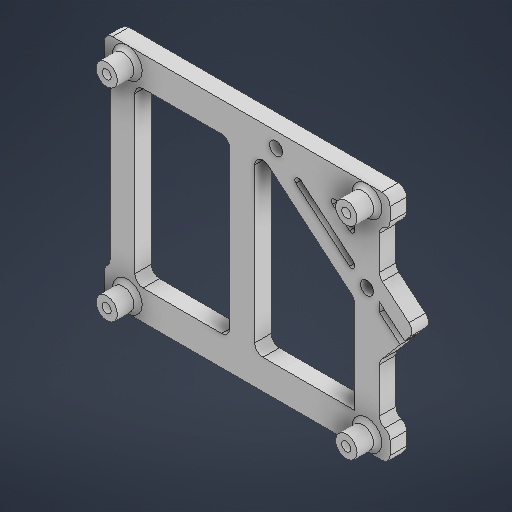
# Autodesk Inventor part: rpi-mount
Saved by Autodesk Inventor 2025 (Build 290162000, 162)
## iProperties
Created: 2024-09-27
Part Number: rpi-mount
Material: Generic
Document SubType Name: Modeling
Designer: Windows 7 was better
Density: 1 g/cm^3
Appearance: Default
Author: Windows 7 was better
Autodesk Inventor part; units mm, degrees
ref_plane "YZ Plane" through (0, 0, 0) normal (1, 0, 0) x (0, 1, 0)
ref_plane "XZ Plane" through (0, 0, 0) normal (0, 1, 0) x (-1, 0, 0)
ref_plane "XY Plane" through (0, 0, 0) normal (0, 0, 1) x (1, 0, 0)
sketch "Sketch1" plane through (0, 0, 0) normal (0, 0, 1) x (1, 0, 0)
  line L0 (0, 0) -> (0, 1.8) construction
  line L1 (-9.2123, 0.9) -> (-9.2123, 25.4) construction
  line L2 (-9.2123, 25.4) -> (-9.2123, -23.6) construction
  line L3 (-9.2123, -23.6) -> (48.7877, -23.6) construction
  line L4 (-9.2123, 25.4) -> (48.7877, 25.4) construction
  circle A0 centre (48.7877, 25.4) radius 1.1
  circle A1 centre (-9.2123, 25.4) radius 1.1
  circle A2 centre (-9.2123, -23.6) radius 1.1
  circle A3 centre (48.7877, -23.6) radius 1.1
  line L5 (-14.8123, -20) -> (54.3877, -20)
  line L6 (54.3877, -20) -> (54.3877, -27.2)
  line L7 (54.3877, -27.2) -> (-14.8123, -27.2)
  line L8 (-14.8123, -27.2) -> (-14.8123, -20)
  line L9 (-14.8123, -20) -> (54.3877, -27.2) construction
  line L10 (54.3877, -20) -> (-14.8123, -27.2) construction
  line L11 (-14.8123, 29) -> (54.3877, 29)
  line L12 (54.3877, 29) -> (54.3877, 21.8)
  line L13 (54.3877, 21.8) -> (-14.8123, 21.8)
  line L14 (-14.8123, 21.8) -> (-14.8123, 29)
  line L15 (-14.8123, 29) -> (54.3877, 21.8) construction
  line L16 (54.3877, 29) -> (-14.8123, 21.8) construction
  line L17 (21.5942, 21.8) -> (15.5942, 21.8)
  line L18 (15.5942, 21.8) -> (15.5942, -20)
  line L19 (15.5942, -20) -> (21.5942, -20)
  line L20 (21.5942, -20) -> (21.5942, 21.8)
  line L21 (-13.4058, 21.8) -> (-7.4058, 21.8)
  line L22 (-7.4058, 21.8) -> (-7.4058, -20)
  line L23 (-7.4058, -20) -> (-13.4058, -20)
  line L24 (-13.4058, -20) -> (-13.4058, 21.8)
  line L25 (19.7877, 25.4) -> (19.7877, 0) construction
  line L26 (48.7877, 25.4) -> (48.7877, -23.6) construction
  line L27 (51.7877, 25.4) -> (51.7877, -23.6)
  line L28 (51.7877, -23.6) -> (45.7877, -23.6)
  line L29 (45.7877, -23.6) -> (45.7877, 25.4)
  line L30 (45.7877, 25.4) -> (51.7877, 25.4)
  line L31 (51.7877, 25.4) -> (45.7877, -23.6) construction
  line L32 (51.7877, -23.6) -> (45.7877, 25.4) construction
  line L33 (54.2512, -3.7837) -> (27.4397, 18.7139)
  line L34 (27.4397, 18.7139) -> (30.0108, 21.7781)
  line L35 (30.0108, 21.7781) -> (56.8224, -0.7195)
  line L36 (56.8224, -0.7195) -> (54.2512, -3.7837)
  line L37 (54.2512, -3.7837) -> (89.2512, -3.7837) construction
  line L38 (30.0108, 21.7781) -> (31.1036, 23.0804) construction
  line L39 (31.1036, 23.0804) -> (57.9151, 0.5828)
  line L40 (57.9151, 0.5828) -> (60.4863, 3.647)
  line L41 (60.4863, 3.647) -> (33.6747, 26.1445)
  line L42 (33.6747, 26.1445) -> (31.1036, 23.0804)
  line L43 (54.2512, -3.7837) -> (45.7877, 3.3181)
  line L44 (47.4017, 0) -> (57.4017, 0) construction
  line L45 (56.8224, -0.7195) -> (57.9151, 0.5828) construction
  line L46 (27.4397, 18.7139) -> (23.7618, 21.8)
  line L47 (54.2512, -3.7837) -> (51.7877, -6.7196)
  line L48 (30.0108, 21.7781) -> (29.9847, 21.8)
  circle A4 centre (48.7877, 7.132) radius 1.6
  circle A5 centre (26.7826, 25.4) radius 1.6
  point P0 (19.7877, -23.6)
  point P1 (15.5942, 21.8)
  point P2 (-13.4058, -20)
  point P3 (21.5942, -20)
  point P4 (48.7877, 0.9)
  point P5 (45.7877, 21.8)
  point P6 (45.7877, -20)
  point P7 (51.7877, -20)
  point P8 (51.7877, 21.8)
  point P9 (45.7877, 15.9806)
  point P10 (38.8523, 21.8)
  point P11 (32.6294, 21.8)
  point P12 (45.7877, 10.7589)
  point P13 (45.7877, 8.5397)
  point P14 (21.5942, 20.2921)
  point P15 (21.5942, 15.0705)
  point P16 (51.7877, 3.5051)
  point P17 (51.7877, -1.7165)
  point P18 (47.6877, -23.6)
  point P19 (49.8877, -23.6)
  point P20 (51.7877, -1.7165)
  point P21 (51.7877, 5.7243)
  point P22 (51.7877, 10.946)
  point P23 (49.8877, 25.4)
  point P24 (47.6877, 25.4)
  dimension "d7" = 24.5
  dimension "d8" = 49
  dimension "d9" = 58
  dimension "d10" = 58
  dimension "d11" = 2.2
  dimension "d12" = 2.2
  dimension "d13" = 2.2
  dimension "d14" = 2.2
  dimension "d15" = 69.2
  dimension "d16" = 7.2
  dimension "d17" = 69.2
  dimension "d18" = 7.2
  dimension "d19" = 6
  dimension "d20" = 6
  dimension "d36" = 6
  dimension "d37" = 35
  dimension "d38" = 140
  dimension "d39" = 4
  dimension "d40" = 1.7
  dimension "d41" = 4
  dimension "d42" = 35
  dimension "d45" = 10
  dimension "d55" = 3.2
  dimension "d56" = 3.2
  constraints: 98 end point, 16 parallel, 11 point on line, 9 midpoint, 9 perpendicular, 8 horizontal, 6 centre point, 4 coincident, 3 vertical, 1 equal length
  measures "d7" distance of L1.start L1.end
  measures "d8" distance of L1.end L2.end
  measures "d9" distance of L2.end L3.end
  measures "d10" distance of L1.end L4.end
  measures "d11" diameter of A0
  measures "d12" diameter of A1
  measures "d13" diameter of A2
  measures "d14" diameter of A3
  measures "d15" distance of L6.end L7.end
  measures "d16" distance of L5.end L6.end
  measures "d17" distance of L12.end L13.end
  measures "d18" distance of L11.end L12.end
  measures "d19" distance of L19.end L18.end
  measures "d20" distance of L22.end L23.end
  measures "d36" distance of L27.end L28.end
  measures "d37" distance of L33.start L33.end
  measures "d38" angle of L37 L33
  measures "d39" distance of L33.end L34.end
  measures "d40" distance of L34.end L38.end
  measures "d41" distance of L40.end L39.end
  measures "d42" distance of L40.end L41.end
  measures "d45" distance of L44.start L44.end
  measures "d55" diameter of A4
  measures "d56" diameter of A5
extrude "Extrusion1" add sketch "Sketch1" along normal blind 4 contours L30 L27 L13 L29 A0 | A0 L30 L29 L13 L41 L42 L39 L14 L11 L12 L27 | L27 L41 L29 L13 | L41 L40 L39 L27 | L27 L39 A4 L29 L41 | L41 L29 L39 L13 | L13 L39 L42 L41 | L27 L35 A4 L39 | L39 A4 L35 L29 | L35 L36 L33 L27 | L27 L33 L29 L35 A4 | L48 L34 L46 L13 | L29 L33 L34 L35 | L33 L47 L27 | L27 L5 L29 L33 | L13 L22 L5 L24 | L20 L5 L18 L13 | L29 L28 A3 L27 L5 L6 L7 L8 | L5 L27 L28 A3 L29
fillet "Fillet5" radius 2 14 edges at (-14.8123, -27.2, 2) (-14.8123, -20, 2) (-13.4058, -20, 2) (-13.4058, 21.8, 2) (-14.8123, 21.8, 2) (-14.8123, 29, 2) (54.3877, 29, 2) (54.3877, 21.8, 2) (54.3877, -20, 2) (54.3877, -27.2, 2) (-7.4058, 21.8, 2) (-7.4058, -20, 2) (15.5942, -20, 2) (21.5942, 21.8, 2)
fillet "Fillet7" radius 2 9 edges at (51.7877, 10.946, 2) (51.7877, -6.7196, 2) (60.4863, 3.647, 2) (51.7877, -20, 2) (51.7877, 21.8, 2) (21.5942, -20, 2) (15.5942, 21.8, 2) (23.7618, 21.8, 2) (45.7877, 3.3181, 2)
fillet "Fillet8" radius 0.75 7 edges at (45.7877, 21.8, 2) (38.8523, 21.8, 2) (45.7877, 15.9806, 2) (32.6294, 21.8, 2) (29.9847, 21.8, 2) (45.7877, 10.7589, 2) (45.7877, 8.5397, 2)
sketch "Sketch3" plane through (0, 0, 4) normal (0, 0, 1) x (1, 0, 0)
  circle A0 centre (-9.2123, 25.4) radius 1.1 projected
  circle A1 centre (48.7877, 25.4) radius 1.1 projected
  circle A2 centre (48.7877, -23.6) radius 1.1 projected
  circle A3 centre (-9.2123, -23.6) radius 1.1 projected
  circle A4 centre (-9.2123, -23.6) radius 2.6
  circle A5 centre (48.7877, -23.6) radius 2.6
  circle A6 centre (48.7877, 25.4) radius 2.6
  circle A7 centre (-9.2123, 25.4) radius 2.6
  point P0 (0, 0)
  dimension "d48" = 1.5
  dimension "d49" = 1.5
  dimension "d50" = 1.5
  dimension "d51" = 1.5
  constraints: 4 centre point
  measures "d48" radial gap between concentric circles of A3 A4
  measures "d49" radial gap between concentric circles of A2 A5
  measures "d50" radial gap between concentric circles of A1 A6
  measures "d51" radial gap between concentric circles of A0 A7
extrude "Extrusion3" add sketch "Sketch3" along normal blind 5
fillet "Fillet9" radius 1 4 edges at (46.1877, 25.4, 4) (46.1877, -23.6, 4) (-11.8123, -23.6, 4) (-11.8123, 25.4, 4)
body "Solid1"
